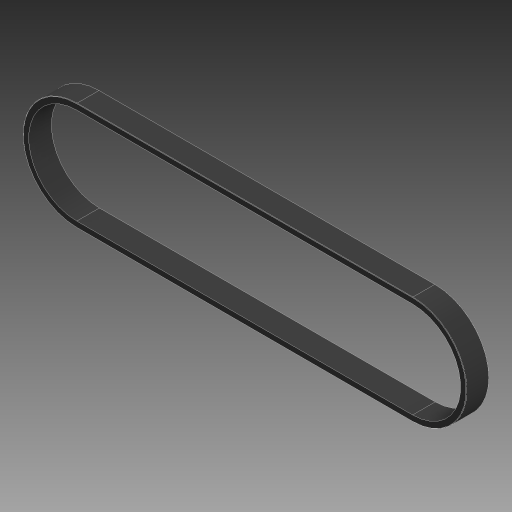
# Autodesk Inventor part: Configurable Kitbot Drive Belt
Saved by Autodesk Inventor 2023 (Build 270158030, 158C)
## iProperties
Created: 2023-01-24
Part Number: Configurable Kitbot Drive Belt
Material: Rubber
Document SubType Name: Modeling
Designer: Max Boord
Density: 0.93 g/cm^3
Appearance: Rubber - Black
Mass: 35.4945 g
Surface Area: 246.611 cm^2
Volume: 38.1661 cm^3
Author: Max Boord
Autodesk Inventor part; units mm, degrees
ref_plane "YZ Plane" through (0, 0, 0) normal (1, 0, 0) x (0, 1, 0)
ref_plane "XZ Plane" through (0, 0, 0) normal (0, 1, 0) x (-1, 0, 0)
ref_plane "XY Plane" through (0, 0, 0) normal (0, 0, 1) x (1, 0, 0)
sketch "Sketch1" plane through (0, 0, 0) normal (0, 0, 1) x (1, 0, 0)
  line L0 (111.25, 0) -> (-111.25, 0) construction
  line L1 (111.25, 33.4225) -> (-111.25, 33.4225) construction
  line L2 (-111.25, -33.4225) -> (111.25, -33.4225) construction
  arc A0 (111.25, -33.4225) -> (111.25, 33.4225) centre (111.25, 0) ccw construction
  arc A1 (-111.25, 33.4225) -> (-111.25, -33.4225) centre (-111.25, 0) ccw construction
  line L3 (-111.25, 35.7085) -> (111.25, 35.7085)
  arc A2 (111.25, -35.7085) -> (111.25, 35.7085) centre (111.25, 0) ccw
  line L4 (111.25, -35.7085) -> (-111.25, -35.7085)
  arc A3 (-111.25, 35.7085) -> (-111.25, -35.7085) centre (-111.25, 0) ccw
  line L5 (-111.25, 31.835) -> (111.25, 31.835)
  arc A4 (111.25, -31.835) -> (111.25, 31.835) centre (111.25, 0) ccw
  line L6 (111.25, -31.835) -> (-111.25, -31.835)
  arc A5 (-111.25, 31.835) -> (-111.25, -31.835) centre (-111.25, 0) ccw
  point P0 (0, 0)
  dimension "d0" = 66.8451
  dimension "d1" = 105
  dimension "d2" = 222.5
  dimension "d3" = 2.286
  dimension "d4" = 1.5875
  constraints: 16 end point, 12 point on circle, 6 centre point, 4 tangent, 3 parallel, 1 horizontal, 1 midpoint, 6 other
  measures "d0" diameter of A1
  measures "d2" distance of L0.start L0.end
  measures "d3" distance between parallel lines of L1 L3
  measures "d4" distance between parallel lines of L1 L5
extrude "Extrusion1" add sketch "Sketch1" along normal mid plane 15
fillet "Fillet1" radius 0.254 8 edges at (0, 35.7085, 7.5) (-146.9585, 0, 7.5) (0, -35.7085, 7.5) (146.9585, 0, 7.5) (146.9585, 0, -7.5) (0, -35.7085, -7.5) (-146.9585, 0, -7.5) (0, 35.7085, -7.5)
body "Solid1"
